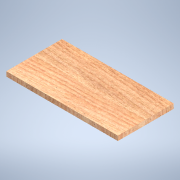
# Autodesk Inventor part: basePlate
Saved by Autodesk Inventor 2020.2 (Build 242310000, 310)
## iProperties
Created: 2020-01-23
Part Number: basePlate
Material: Wood (Birch)
Document SubType Name: Modeling
Designer: robst
Density: 0.55 g/cm^3
Appearance: Birch - Natural Polished
Author: robst
Autodesk Inventor part; units mm, degrees
ref_plane "YZ Plane" through (0, 0, 0) normal (1, 0, 0) x (0, 1, 0)
ref_plane "XZ Plane" through (0, 0, 0) normal (0, 1, 0) x (-1, 0, 0)
ref_plane "XY Plane" through (0, 0, 0) normal (0, 0, 1) x (1, 0, 0)
sketch "Sketch1" plane through (0, 0, 0) normal (0, 1, 0) x (-1, 0, 0)
  line L0 (152.4, 76.2) -> (-152.4, 76.2)
  line L1 (-152.4, 76.2) -> (-152.4, -76.2)
  line L2 (-152.4, -76.2) -> (152.4, -76.2)
  line L3 (152.4, -76.2) -> (152.4, 76.2)
  line L4 (152.4, 76.2) -> (-152.4, -76.2) construction
  line L5 (-152.4, 76.2) -> (152.4, -76.2) construction
  point P0 (0, 0)
  dimension "d0" = 304.8
  dimension "d1" = 152.4
  constraints: 12 end point, 2 midpoint, 2 parallel, 1 horizontal, 1 perpendicular
  measures "d0" distance of L0.start L0.end
  measures "d1" distance of L1.end L0.end
extrude "Extrusion1" add sketch "Sketch1" against normal blind 12.7
sketch "Sketch2" plane through (0, 0, 0) normal (0, 1, 0) x (1, 0, 0)
  line L0 (-152.4, 76.2) -> (-152.4, -76.2) construction
  line L1 (152.4, -76.2) -> (152.4, 76.2) construction
  line L2 (-152.4, -76.2) -> (-152.4, 76.2) construction
  line L3 (-152.4, 31.75) -> (152.4, 31.75) construction
  line L4 (152.4, 76.2) -> (152.4, -76.2) construction
  line L5 (152.4, 76.2) -> (-152.4, 76.2) construction
  line L6 (-101.6, 31.75) -> (-101.6, 76.2) construction
  line L7 (101.6, 31.75) -> (101.6, 76.2) construction
  point P0 (0, 0)
  dimension "centerLineForAirTank" = 44.45
  dimension "distanceFromEndForAirTankBracket" = 50.8
  dimension "d6" = 50.8
  constraints: 6 end point, 6 point on line, 2 perpendicular, 1 vertical
  measures "centerLineForAirTank" distance between parallel lines of L5 L3
  measures "distanceFromEndForAirTankBracket" distance from line of L0 L6.start
  measures "d6" distance from line of L1 L7.start
hole "Hole1" at (-101.6, 0, -31.75) at (101.6, 0, -31.75) direction (0, -1, 0) diameter 5.1054 end through all clearance for "Hex Machine Screw" size "#10" standard "Ansi Unified Screw Threads"
equation "\"d6\" = distanceFromEndForAirTankBracket"
body "Solid1"
